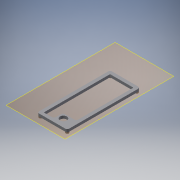
# Autodesk Inventor part: 31_Handyaufnahme_2
Saved by Autodesk Inventor 2016 (Build 200138000, 138)
## iProperties
Created: 2016-09-16
Part Number: 31_Handyaufnahme_2
Material: Generisch
Document SubType Name: Modeling
Designer: Bene
Density: 1 g/cm^3
Appearance: Vorgabe
Author: Bene
Autodesk Inventor part; units mm, degrees
ref_plane "YZ Plane" through (0, 0, 0) normal (1, 0, 0) x (0, 1, 0)
ref_plane "XZ Plane" through (0, 0, 0) normal (0, 1, 0) x (-1, 0, 0)
ref_plane "XY Plane" through (0, 0, 0) normal (0, 0, 1) x (1, 0, 0)
ref_plane "Arbeitsebene1" through (0, 0, 0) normal (0, 0, 1) x (1, 0, 0)
sketch "Skizze1" plane through (0, 0, 0) normal (0, 0, 1) x (1, 0, 0)
  arc A0 (37.0113, -74.16) -> (40.0113, -71.16) centre (37.0113, -71.16) ccw construction
  line L0 (40.0113, -71.16) -> (40.0113, 71.16) construction
  arc A1 (40.0113, 71.16) -> (37.0113, 74.16) centre (37.0113, 71.16) ccw construction
  line L1 (37.0113, 74.16) -> (-37.0113, 74.16) construction
  arc A2 (-37.0113, 74.16) -> (-40.0113, 71.16) centre (-37.0113, 71.16) ccw construction
  line L2 (-40.0113, 71.16) -> (-40.0113, -71.16) construction
  arc A3 (-40.0113, -71.16) -> (-37.0113, -74.16) centre (-37.0113, -71.16) ccw construction
  line L3 (-37.0113, -74.16) -> (37.0113, -74.16) construction
  circle A4 centre (-5, -69.16) radius 2.5 construction
  circle A5 centre (35.0113, 35.0572) radius 2.5 construction
  circle A6 centre (35.0113, -69.16) radius 2.5 construction
  circle A7 centre (-5, 35.0572) radius 2.5 construction
  circle A8 centre (20, -59.8179) radius 9.5 construction
  circle A9 centre (20, -59.8179) radius 1 construction
  line L4 (15.25, -57.8504) -> (18.0325, -55.0679) construction
  line L5 (18.0325, -55.0679) -> (21.9675, -55.0679) construction
  line L6 (21.9675, -55.0679) -> (24.75, -57.8504) construction
  line L7 (24.75, -57.8504) -> (24.75, -61.7854) construction
  line L8 (24.75, -61.7854) -> (21.9675, -64.5679) construction
  line L9 (21.9675, -64.5679) -> (18.0325, -64.5679) construction
  line L10 (18.0325, -64.5679) -> (15.25, -61.7854) construction
  line L11 (15.25, -61.7854) -> (15.25, -57.8504) construction
  line L12 (37.5113, -71.66) -> (-7.5, -71.66)
  line L13 (-7.5, -71.66) -> (-7.5, -66.66)
  line L14 (-7.5, -66.66) -> (37.5113, -66.66)
  line L15 (37.5113, -66.66) -> (37.5113, -71.66)
  line L16 (-7.5, -71.66) -> (-2.5, -71.66)
  line L17 (-2.5, -71.66) -> (-2.5, 37.5572)
  line L18 (-2.5, 37.5572) -> (-7.5, 37.5572)
  line L19 (-7.5, 37.5572) -> (-7.5, -71.66)
  line L20 (-7.5, 37.5572) -> (37.5113, 37.5572)
  line L21 (37.5113, 37.5572) -> (37.5113, 32.5572)
  line L22 (37.5113, 32.5572) -> (-7.5, 32.5572)
  line L23 (-7.5, 32.5572) -> (-7.5, 37.5572)
  line L24 (37.5113, 37.5572) -> (32.5113, 37.5572)
  line L25 (32.5113, 37.5572) -> (32.5113, -71.66)
  line L26 (32.5113, -71.66) -> (37.5113, -71.66)
  line L27 (37.5113, -71.66) -> (37.5113, 37.5572)
  point P0 (0, 0)
  point P1 (-2.5, 32.5572)
  point P2 (32.5113, 32.5572)
  point P3 (32.5113, -66.66)
  point P4 (-2.5, -66.66)
  constraints: 32 end point, 10 point on line, 8 parallel, 4 horizontal, 4 perpendicular
extrude "Extrusion1" add sketch "Skizze1" along normal blind 4 contours L12 L25 L14 L15 | L12 L17 L14 L25 | L14 L25 L22 L27 | L12 L13 L14 L17 | L22 L25 L20 L21 | L14 L19 L22 L17 | L22 L17 L20 L25 | L22 L19 L18 L17
sketch "Skizze2" plane through (0, 0, 4) normal (0, 0, 1) x (1, 0, 0)
  line L0 (15.25, -61.7854) -> (15.25, -57.8504) construction
  line L1 (18.0325, -64.5679) -> (15.25, -61.7854) construction
  line L2 (21.9675, -64.5679) -> (18.0325, -64.5679) construction
  line L3 (24.75, -61.7854) -> (21.9675, -64.5679) construction
  line L4 (24.75, -57.8504) -> (24.75, -61.7854) construction
  line L5 (21.9675, -55.0679) -> (24.75, -57.8504) construction
  line L6 (18.0325, -55.0679) -> (21.9675, -55.0679) construction
  line L7 (15.25, -57.8504) -> (18.0325, -55.0679) construction
  line L8 (32.5113, -66.66) -> (-2.5, -66.66) projected
  line L9 (-2.5, -66.66) -> (-2.5, 32.5572) projected
  line L10 (-2.5, 32.5572) -> (32.5113, 32.5572) projected
  line L11 (32.5113, 32.5572) -> (32.5113, -66.66) projected
  line L12 (-7.5, -71.66) -> (37.5113, -71.66) projected
  line L13 (37.5113, -71.66) -> (37.5113, 37.5572) projected
  line L14 (37.5113, 37.5572) -> (-7.5, 37.5572) projected
  line L15 (-7.5, 37.5572) -> (-7.5, -71.66) projected
  circle A0 centre (20, -59.8179) radius 5.1414
  line L16 (32.5113, -66.66) -> (-2.5, -66.66) projected
  line L17 (32.5113, -66.66) -> (12.5113, -66.66)
  line L18 (12.5113, -66.66) -> (12.5113, -53.16)
  line L19 (12.5113, -53.16) -> (32.5113, -53.16)
  line L20 (32.5113, -53.16) -> (32.5113, -66.66)
  point P0 (0, 0)
  dimension "d2" = 20
  dimension "d3" = 13.5
  constraints: 8 end point, 2 parallel, 1 horizontal, 1 perpendicular, 3 other
  measures "d2" distance of L18.end L19.end
  measures "d3" distance of L17.end L18.end
extrude "Extrusion2" add sketch "Skizze2" against normal up to surface (4 mm away) contours L8 L18 L19 L11
sketch "Skizze5" plane through (0, 0, 0) normal (0, 0, -1) x (-1, 0, 0)
  circle A0 centre (5, -69.16) radius 2.5 construction
  circle A1 centre (5, 35.0572) radius 2.5 construction
  circle A2 centre (-35.0113, 35.0572) radius 2.5 construction
  arc A3 (-37.5, -69.3969) -> (-37.5, -68.923) centre (-35.0113, -69.16) ccw construction
  circle A4 centre (-35.0113, 35.0572) radius 2.4
  circle A5 centre (5, 35.0572) radius 2.4
  circle A6 centre (5, -69.16) radius 2.4
  circle A7 centre (-35.0113, -69.16) radius 2.4
  point P0 (0, 0)
  dimension "d13" = 4.8
  dimension "d14" = 4.8
  dimension "d15" = 4.8
  dimension "d16" = 4.8
  constraints: 4 centre point, 4 coincident
  measures "d13" diameter of A4
  measures "d14" diameter of A5
  measures "d15" diameter of A6
  measures "d16" diameter of A7
extrude "Extrusion4" add sketch "Skizze5" along normal blind 2
fillet "Rundung1" radius 3 7 edges at (-7.5, -71.66, 2) (37.5113, -71.66, 2) (37.5113, 37.5572, 2) (-7.5, 37.5572, 2) (12.5113, -66.66, 2) (12.5113, -53.16, 2) (32.5113, -53.16, 2)
